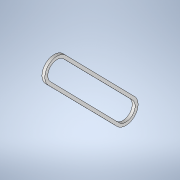
# Autodesk Inventor part: belt
Saved by Autodesk Inventor 2021 (Build 250183000, 183)
## iProperties
Created: 2021-04-10
Part Number: belt
Material: Generic
Document SubType Name: Modeling
Designer: deli
Density: 1 g/cm^3
Appearance: Default
Author: deli
Autodesk Inventor part; units mm, degrees
ref_plane "YZ Plane" through (0, 0, 0) normal (1, 0, 0) x (0, 1, 0)
ref_plane "XZ Plane" through (0, 0, 0) normal (0, 1, 0) x (-1, 0, 0)
ref_plane "XY Plane" through (0, 0, 0) normal (0, 0, 1) x (1, 0, 0)
sketch "Sketch1" plane through (0, 0, 0) normal (1, 0, 0) x (0, 1, 0)
  circle A0 centre (-10.828, 28.2084) radius 15.975 projected
  circle A1 centre (108.9876, 145.8935) radius 16
  line L0 (0.3646, 16.8099) -> (120.1977, 134.4771)
  line L1 (-22.0239, 39.6037) -> (97.7741, 157.3065)
  circle A2 centre (-10.828, 28.2084) radius 20.975
  line L2 (-25.5281, 43.1703) -> (94.2699, 160.8731)
  line L3 (3.8677, 13.2422) -> (123.7008, 130.9094)
  circle A3 centre (108.9876, 145.8935) radius 21
  point P0 (0, 0)
  dimension "d0" = 5
  dimension "d1" = 5
  dimension "d2" = 5
  dimension "d3" = 5
  constraints: 8 end point, 4 point on circle, 4 tangent, 3 centre point, 2 parallel, 2 other
  measures "d0" radial gap between concentric circles of A0 A2
  measures "d1" distance between parallel lines of L1 L2
  measures "d2" distance between parallel lines of L0 L3
  measures "d3" radial gap between concentric circles of A1 A3
extrude "Extrusion1" add sketch "Sketch1" along normal blind 5 contours A0 L0 A2 L1 | A2 L2 A3 L1 | L0 A3 L3 A2 | A3 L0 A1 L1 picked at (6.4932, 21.5544) picked at (91.6433, 152.5567)
fillet "Fillet1" radius 2.5 16 edges at (0, -25.792, 13.5105) (0, 63.7843, 72.0758) (0, 123.9694, 160.6089) (0, 34.3709, 102.0217) (5, -25.792, 13.5105) (5, 63.7843, 72.0758) (5, 123.9694, 160.6089) (5, 34.3709, 102.0217) (5, 120.4023, 157.1052) (5, 60.2811, 75.6435) (5, -22.2249, 17.0142) (5, 37.8751, 98.4551) (0, -22.2249, 17.0142) (0, 37.8751, 98.4551) (0, 120.4023, 157.1052) (0, 60.2811, 75.6435)
body "Solid1"
